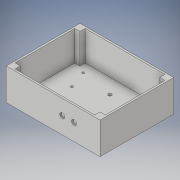
# Autodesk Inventor part: 546-1590BBS-ADF4360-9
Saved by Autodesk Inventor 2018 (Build 220112000, 112)
## iProperties
Created: 2018-04-27
Part Number: 546-1590BBS-ADF4360-9
Material: Generic
Document SubType Name: Modeling
Designer: bbramman
Density: 1 g/cm^3
Appearance: Default
Author: bbramman
Autodesk Inventor part; units mm, degrees
ref_plane "YZ Plane" through (0, 0, 0) normal (1, 0, 0) x (0, 1, 0)
ref_plane "XZ Plane" through (0, 0, 0) normal (0, 1, 0) x (-1, 0, 0)
ref_plane "XY Plane" through (0, 0, 0) normal (0, 0, 1) x (1, 0, 0)
sketch "Sketch1" plane through (0, 0, 0) normal (0, 1, 0) x (-1, 0, 0)
  line L0 (-59.7535, -47.0027) -> (59.7535, -47.0027)
  line L1 (59.7535, -47.0027) -> (59.7535, 47.0027)
  line L2 (59.7535, 47.0027) -> (-59.7535, 47.0027)
  line L3 (-59.7535, 47.0027) -> (-59.7535, -47.0027)
  line L4 (-59.7535, -47.0027) -> (59.7535, 47.0027) construction
  line L5 (59.7535, -47.0027) -> (-59.7535, 47.0027) construction
  point P0 (0, 0)
  dimension "d0" = 119.507
  dimension "d1" = 94.0054
  constraints: 12 end point, 2 midpoint, 2 parallel, 1 horizontal, 1 perpendicular
  measures "d0" distance of L2.end L1.end
  measures "d1" distance of L1.end L0.end
extrude "Extrusion1" add sketch "Sketch1" along normal mid plane 2.2606
sketch "Sketch2" plane through (0, 1.1303, 0) normal (0, 1, 0) x (1, 0, 0)
  line L0 (-59.7535, 47.0027) -> (-59.7535, -47.0027) projected
  line L1 (59.7535, -47.0027) -> (59.7535, 47.0027) projected
  line L2 (-59.7535, -47.0027) -> (59.7535, -47.0027)
  line L3 (59.7535, -47.0027) -> (59.7535, 47.0027)
  line L4 (59.7535, 47.0027) -> (-59.7535, 47.0027)
  line L5 (-59.7535, 47.0027) -> (-59.7535, -47.0027)
  line L6 (57.4929, -44.7421) -> (-57.4929, 44.7421) construction
  line L7 (-57.4929, -44.7421) -> (57.4929, 44.7421) construction
  line L8 (-59.7535, -47.0027) -> (59.7535, -47.0027) projected
  line L9 (-59.7535, -47.0027) -> (-50.7619, -47.0027)
  line L10 (-59.7535, -38.0111) -> (-59.7535, -47.0027)
  line L11 (-59.7535, 47.0027) -> (-50.7619, 47.0027)
  line L12 (-59.7535, 38.0111) -> (-59.7535, 47.0027)
  line L13 (59.7535, 47.0027) -> (-59.7535, 47.0027) projected
  line L14 (59.7535, 47.0027) -> (50.7619, 47.0027)
  line L15 (59.7535, 38.0111) -> (59.7535, 47.0027)
  line L16 (59.7535, -47.0027) -> (50.7619, -47.0027)
  line L17 (59.7535, -38.0111) -> (59.7535, -47.0027)
  line L18 (-50.7619, -44.7421) -> (-50.7619, -38.0111)
  line L19 (-50.7619, -38.0111) -> (-57.4929, -38.0111)
  line L20 (-57.4929, 38.0111) -> (-50.7619, 38.0111)
  line L21 (-50.7619, 38.0111) -> (-50.7619, 44.7421)
  line L22 (50.7619, 38.0111) -> (57.4929, 38.0111)
  line L23 (50.7619, 44.7421) -> (50.7619, 38.0111)
  line L24 (57.4929, -38.0111) -> (50.7619, -38.0111)
  line L25 (50.7619, -38.0111) -> (50.7619, -44.7421)
  line L26 (-50.7619, -44.7421) -> (50.7619, -44.7421)
  line L27 (57.4929, -38.0111) -> (57.4929, 38.0111)
  line L28 (50.7619, 44.7421) -> (-50.7619, 44.7421)
  line L29 (-57.4929, 38.0111) -> (-57.4929, -38.0111)
  point P0 (0, 0)
  dimension "d4" = 114.9858
  dimension "d5" = 89.4842
  dimension "d6" = 8.9916
  dimension "d7" = 8.9916
  dimension "d10" = 8.9916
  dimension "d11" = 8.9916
  constraints: 52 end point, 7 horizontal, 3 perpendicular, 2 midpoint, 2 parallel
  measures "d4" distance of L6.end L7.end
  measures "d5" distance of L7.start L6.end
  measures "d6" distance of L10.start L18.end
  measures "d7" distance of L18.end L9.end
  measures "d10" distance of L15.start L22.start
  measures "d11" distance of L22.start L14.end
extrude "Extrusion2" add sketch "Sketch2" along normal blind 38.1
sketch "Sketch3" plane through (0, 1.1303, 0) normal (0, 1, 0) x (1, 0, 0)
  circle A0 centre (0, -25.4) radius 2.0828
  circle A1 centre (0, 25.4) radius 2.0828
  point P0 (0, 0)
  dimension "d18" = 4.1656
  dimension "d19" = 4.1656
  constraints: 2 centre point
  measures "d18" diameter of A0
  measures "d19" diameter of A1
extrude "Extrusion3" cut sketch "Sketch3" against normal through all
sketch "Sketch7" plane through (0, 1.1303, 0) normal (0, 1, 0) x (1, 0, 0)
  line L0 (32.9946, -9.9949) -> (-32.9946, 9.9949) construction
  line L1 (-32.9946, -9.9949) -> (32.9946, 9.9949) construction
  circle A0 centre (-32.9946, -9.9949) radius 1.4986
  circle A1 centre (-32.9946, 9.9949) radius 1.4986
  circle A2 centre (32.9946, 9.9949) radius 1.4986
  circle A3 centre (32.9946, -9.9949) radius 1.4986
  line L2 (47.498, -29.9974) -> (-47.498, 29.9974) construction
  line L3 (-47.498, -29.9974) -> (47.498, 29.9974) construction
  line L4 (-47.498, 29.9974) -> (-41.148, 29.9974) construction
  line L5 (47.498, 29.9974) -> (53.848, 29.9974) construction
  circle A4 centre (-41.148, -32.5374) radius 1.4224
  circle A5 centre (41.148, -32.5374) radius 1.4224
  circle A6 centre (41.148, 32.5374) radius 1.4224
  circle A7 centre (-41.148, 32.5374) radius 1.4224
  point P0 (0, 0)
  dimension "d48" = 19.9898
  dimension "d49" = 2.9972
  dimension "d50" = 2.9972
  dimension "d51" = 2.9972
  dimension "d52" = 2.9972
  dimension "d65" = 2.8448
  dimension "d66" = 2.8448
  dimension "d68" = 2.8448
  constraints: 12 end point, 8 centre point, 4 coincident, 4 midpoint, 2 horizontal
  measures "d48" distance of L1.start L0.end
  measures "d49" diameter of A0
  measures "d50" diameter of A1
  measures "d51" diameter of A2
  measures "d52" diameter of A3
  measures "d65" diameter of A4
  measures "d66" diameter of A5
  measures "d68" diameter of A7
extrude "Extrusion6" cut sketch "Sketch7" against normal through all
sketch "Sketch8" plane through (50.7619, 1.1303, 44.7421) normal (0, 0, -1) x (-1, 0, 0)
  circle A0 centre (23.9014, 19.05) radius 3.175
  circle A1 centre (38.989, 19.05) radius 3.175
  point P0 (50.7619, -1.1303)
  dimension "d74" = 6.35
  dimension "d75" = 6.35
  constraints: 2 centre point
  measures "d74" diameter of A0
  measures "d75" diameter of A1
extrude "Extrusion7" cut sketch "Sketch8" against normal through all
body "Solid1"
